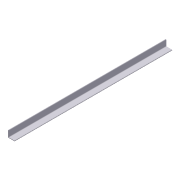
# Autodesk Inventor part: FE-00005-01
Saved by Autodesk Inventor 2012 (Build 160160000, 160)
## iProperties
Company: FIRST
Created: 2008-05-25
Part Number: FE-00005-01
Document SubType Name: Modeling
Designer: dfoster
Density: 1 g/cm^3
Description: Bottom Rail, Field Rail
Mass: 1682.71 g
Surface Area: 5447.04 cm^2
Volume: 1682.71 cm^3
Material: Default
Title: Bottom Rail, Field Rail
Author: dfoster
Autodesk Inventor part; units mm, degrees
ref_plane "YZ Plane" through (0, 0, 0) normal (1, 0, 0) x (0, 1, 0)
ref_plane "XZ Plane" through (0, 0, 0) normal (0, 1, 0) x (-1, 0, 0)
ref_plane "XY Plane" through (0, 0, 0) normal (0, 0, 1) x (1, 0, 0)
sketch "Sketch1" plane through (0, 0, 0) normal (0, 0, 1) x (1, 0, 0)
  line L0 (-32.4184, 42.5283) -> (-32.4184, -33.6717)
  line L1 (-32.4184, -33.6717) -> (43.7816, -33.6717)
  line L2 (43.7816, -33.6717) -> (43.7816, -33.4177)
  line L3 (37.6856, -27.3217) -> (-19.7184, -27.3217)
  line L4 (-26.0684, -20.9717) -> (-26.0684, 36.4323)
  line L5 (-32.1644, 42.5283) -> (-32.4184, 42.5283)
  arc A0 (-26.0684, 36.4323) -> (-32.1644, 42.5283) centre (-32.1644, 36.4323) ccw
  arc A1 (43.7816, -33.4177) -> (37.6856, -27.3217) centre (37.6856, -33.4177) ccw
  arc A2 (-26.0684, -20.9717) -> (-19.7184, -27.3217) centre (-19.7184, -20.9717) ccw
  dimension "d0" = 76.2
  dimension "d1" = 6.096
  dimension "d2" = 6.35
  dimension "d3" = 6.35
  constraints: 12 end point, 6 point on circle, 6 tangent, 4 parallel, 3 centre point, 3 perpendicular, 1 equal radius, 1 vertical
  measures "d0" distance of L0.start L0.end
  measures "d1" radius of A0
  measures "d2" distance between parallel lines of L4 L0
  measures "d3" radius of A2
extrude "Extrusion1" add sketch "Sketch1" along normal blind 1828.8
body "Solid1"
